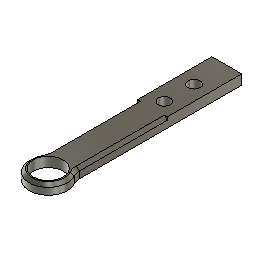
UCF_CutterMount (Autodesk Fusion 360 design; units mm, degrees)
Autodesk Fusion 360 part; units mm, degrees
note: some values were not read from the file. Chosen so that the rebuilt part matches the saved one: which bodies a step acts on; which face or edge a step refers to. Set by a fixed rule: which sketch regions a step uses.
sketch "Sketch1" plane through (0, 0, 0) normal (0, 0, 1) x (1, 0, 0) in component "CutterMount"
  circle A0 centre (0, 0) radius 6.35
  line L0 (-6.35, 6.9514) -> (-6.35, 76.2)
  line L1 (0, 0) -> (0, 76.2) construction
  line L2 (6.35, 6.9514) -> (6.35, 76.2)
  line L3 (-6.35, 76.2) -> (6.35, 76.2)
  arc A1 (-7.1298, 3.9026) -> (7.1298, 3.9026) centre (0, 0) ccw
  circle A2 centre (0, 62.23) radius 2.54
  circle A3 centre (0, 49.53) radius 2.54
  line L4 (-6.35, 44.45) -> (6.35, 44.45)
  arc A4 (6.35, 6.9514) -> (7.1298, 3.9026) centre (12.7, 6.9514) ccw
  arc A5 (-7.1298, 3.9026) -> (-6.35, 6.9514) centre (-12.7, 6.9514) ccw
  dimension "d13_1" = 12.7
  dimension "d16_1" = 6.35
  dimension "d17_1" = 76.2
  dimension "d18_1" = 8.128
  dimension "d19_1" = 5.08
  dimension "d20_1" = 5.08
  dimension "d21_1" = 12.7
  dimension "d198_1" = 13.97
  dimension "d1" = 31.75
  dimension "d2" = 6.35
  constraint coincident A0.centre L1.start
  constraint vertical L0
  constraint parallel L0 L1
  constraint symmetric L0.end L1 L2.end
  constraint coincident L1.end L3
  constraint concentric A0 A1
  constraint coincident L1 A2.centre
  constraint coincident L1 A3.centre
  constraint coincident L0 L4.start
  constraint coincident L2 L4.end
  constraint tangent A1 A4
  constraint tangent L2 A4
  constraint tangent L0 A5
  constraint tangent A1 A5
  constraint equal A4 A5
  measures "d13_1" diameter of A0
  measures "d16_1" distance of A0.centre L0
  measures "d17_1" distance of A0.centre L1.end
  measures "d18_1" radius of A1
  measures "d19_1" diameter of A2
  measures "d20_1" diameter of A3
  measures "d21_1" distance of A2.centre A3.centre
  measures "d198_1" distance of L3 A2.centre
  measures "d2" radius of A4
extrude "Extrude1" add sketch "Sketch1" against normal blind 4.1783 makes body 1 in component "CutterMount"
split "Split2" by curves path "Sketch1" along L4 bodies 1 makes body 2 at (0.1582, 31.7441, 0) in component "CutterMount"
chamfer "Chamfer3" distance 1.27 angle 45 5 edges at (6.35, 25.7007, 0) (6.548, 5.3779, 0) (0, -8.128, 0) (-6.548, 5.3779, 0) (-6.35, 25.7007, 0) on bodies 2 in component "CutterMount"
combine "Combine2" operation add target body 2 tool bodies 1 in component "CutterMount"
component "CutterMount" placed x (1, 0, 0) y (0, 1, 0) z (0, 0, 1) at (0, 0, 0)
